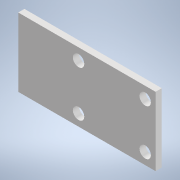
# Autodesk Inventor part: Part21
Saved by Autodesk Inventor 2020.2 (Build 242310000, 310)
## iProperties
Created: 2022-11-16
Part Number: Part21
Material: 一般
Document SubType Name: Modeling
Designer: Administrator
Density: 1 g/cm^3
Appearance: 既定
Author: Administrator
Autodesk Inventor part; units mm, degrees
ref_plane "YZ Plane" through (0, 0, 0) normal (1, 0, 0) x (0, 1, 0)
ref_plane "XZ Plane" through (0, 0, 0) normal (0, 1, 0) x (-1, 0, 0)
ref_plane "XY Plane" through (0, 0, 0) normal (0, 0, 1) x (1, 0, 0)
sketch "スケッチ1" plane through (0, 0, 0) normal (0, 0, 1) x (1, 0, 0)
  circle A0 centre (-1074.3962, 331.6958) radius 2.75
  line L0 (-1069.3962, 326.1958) -> (-1069.3962, 337.1958)
  line L1 (-1083.3962, 337.1958) -> (-1069.3962, 337.1958)
  line L2 (-1083.3962, 326.1958) -> (-1083.3962, 337.1958)
  line L3 (-1069.3962, 326.1958) -> (-1083.3962, 326.1958)
  circle A1 centre (-1074.3962, 309.6958) radius 2.75
  line L4 (-1069.3962, 304.1958) -> (-1069.3962, 315.1958)
  line L5 (-1083.3962, 315.1958) -> (-1069.3962, 315.1958)
  line L6 (-1083.3962, 304.1958) -> (-1083.3962, 315.1958)
  line L7 (-1069.3962, 304.1958) -> (-1083.3962, 304.1958)
  circle A2 centre (-1106.3962, 309.6958) radius 2.75
  line L8 (-1097.3962, 304.1958) -> (-1097.3962, 315.1958)
  line L9 (-1111.3962, 315.1958) -> (-1097.3962, 315.1958)
  line L10 (-1111.3962, 304.1958) -> (-1111.3962, 315.1958)
  line L11 (-1097.3962, 304.1958) -> (-1111.3962, 304.1958)
  circle A3 centre (-1106.3962, 331.6958) radius 2.75
  line L12 (-1097.3962, 326.1958) -> (-1097.3962, 337.1958)
  line L13 (-1111.3962, 337.1958) -> (-1097.3962, 337.1958)
  line L14 (-1111.3962, 326.1958) -> (-1111.3962, 337.1958)
  line L15 (-1097.3962, 326.1958) -> (-1111.3962, 326.1958)
  line L16 (-1064.3962, 273.1958) -> (-1044.3962, 273.1958)
  circle A4 centre (-1054.3962, 265.1958) radius 4.5
  line L17 (-1064.3962, 283.1958) -> (-1044.3962, 283.1958)
  line L18 (-1044.3962, 257.1958) -> (-1044.3962, 283.1958)
  line L19 (-1064.3962, 257.1958) -> (-1044.3962, 257.1958)
  line L20 (-1064.3962, 283.1958) -> (-1064.3962, 257.1958)
  circle A5 centre (-1054.3962, 329.1958) radius 4.5
  line L21 (-1064.3962, 337.1958) -> (-1044.3962, 337.1958)
  line L22 (-1044.3962, 311.1958) -> (-1044.3962, 337.1958)
  line L23 (-1064.3962, 311.1958) -> (-1044.3962, 311.1958)
  line L24 (-1064.3962, 337.1958) -> (-1064.3962, 311.1958)
  line L25 (-1111.3962, 337.1958) -> (-1044.3962, 337.1958)
  line L26 (-1111.3962, 337.1958) -> (-1111.3962, 304.1958)
  line L27 (-1064.3962, 257.1958) -> (-1111.3962, 304.1958)
  line L28 (-1044.3962, 337.1958) -> (-1044.3962, 257.1958)
  line L29 (-1044.3962, 257.1958) -> (-1064.3962, 257.1958)
  point P0 (0, 0)
  point P1 (-1059.3962, 337.1958)
  point P2 (-1064.3962, 337.1958)
extrude "押し出し1" add sketch "スケッチ1" along normal blind 3 contours L3 L2 L1 L0 | L0 L25 L24 L23 L28 L17 L20 L27 L11 L8 L9 L26 L15 L12 L2 L3 | L21 L22 L23 L24 | L12 L15 L14 L13 | L18 L16 L20 L17 | L9 L8 L11 L10 | L18 L19 L20 L16 | L7 L6 L5 L4
